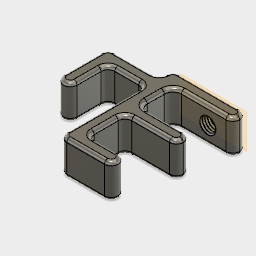
Clamp-Hooks (Autodesk Fusion 360 design; units mm, degrees)
Autodesk Fusion 360 part; units mm, degrees
sketch "Sketch1" plane through (0, 0, 0) normal (0, 1, 0) x (1, 0, 0)
  line L0 (-5, 15) -> (30, 15)
  line L1 (30, 15) -> (30, -5)
  line L2 (30, -5) -> (-5, -5)
  line L3 (-5, -5) -> (-5, 15)
  line L4 (30, 23) -> (-13, 23)
  line L5 (-13, 23) -> (-13, -13)
  line L6 (-13, -13) -> (30, -13)
  line L7 (30, -13) -> (30, 23)
  line L8 (-13, -13) -> (-49, -13)
  line L9 (-49, -13) -> (-49, 23)
  line L10 (-49, 23) -> (-13, 23)
  line L11 (-13, 23) -> (-13, -13)
  line L12 (30, -5) -> (25, -5)
  line L13 (25, -5) -> (25, -13)
  line L14 (25, -13) -> (30, -13)
  line L15 (30, -13) -> (30, -5)
  dimension "d7" = 36
  dimension "d21" = 8
  dimension "d22" = 5
  constraint horizontal L0
  constraint vertical L1
  constraint horizontal L2
  constraint vertical L3
  constraint horizontal L4
  constraint vertical L5
  constraint horizontal L6
  constraint vertical L7
  constraint horizontal L8
  constraint vertical L9
  constraint horizontal L10
  constraint vertical L11
  constraint horizontal L12
  constraint vertical L13
  constraint horizontal L14
  constraint vertical L15
  measures "d7" distance of origin
  measures "d21" distance of origin
extrude "Extrude1" add sketch "Sketch1" along normal blind 20 contours L0 L2 L3 L4 L5 L6 L7 L11 L13 | L2 L6 L7 L12 L13 L14 L15
fillet "Fillet2" radius 5 2 edges at (-5, 10, 5) (-5, 10, -15)
sketch "Sketch2" plane through (0, 0, -15) normal (0, 0, 1) x (1, 0, 0)
  line L0 (0, 20) -> (0, 0)
  line L1 (0, 0) -> (30, 0)
  line L2 (30, 0) -> (30, 20)
  line L3 (30, 20) -> (0, 20)
  circle A0 centre (15, 10) radius 5
extrude "Extrude2" cut sketch "Sketch2" against normal blind 10 contours A0
thread "Thread1" "ISO Metric profile 10.0 M10x1.5 6H" major diameter 10.198 minor diameter 8.526 pitch 1.5 angle 60 modelled right hand crest width 0.1875 on face at (19.9752, 9.5022, -17.6667) crest through (19.263, 10, -14.1562)
sketch "Sketch5" plane through (0, 0, 0) normal (0, -1, 0) x (1, 0, 0)
  line L0 (30, 5) -> (30, 13)
  line L1 (30, 13) -> (-13, 13)
  line L2 (-13, 13) -> (-13, -23)
  line L3 (-13, -23) -> (30, -23)
  line L4 (30, -23) -> (30, -15)
  line L5 (30, -15) -> (0, -15)
  arc A0 (-5, -10) -> (0, -15) centre (0, -10) ccw
  line L6 (-5, -10) -> (-5, 0)
  arc A1 (0, 5) -> (-5, 0) centre (0, 0) ccw
  line L7 (0, 5) -> (30, 5)
  line L8 (-13, -15) -> (-43, -15)
  line L9 (-43, -15) -> (-43, 15)
  line L10 (-43, 15) -> (-13, 15)
  line L11 (-13, 15) -> (-13, -15)
  line L12 (-13, 15) -> (-35, 15)
  line L13 (-35, 15) -> (-35, -7)
  line L14 (-35, -7) -> (-13, -7)
  line L15 (-13, -7) -> (-13, 15)
  line L16 (-13, 13) -> (17, 13)
  line L17 (17, 13) -> (17, 43)
  line L18 (17, 43) -> (-13, 43)
  line L19 (-13, 43) -> (-13, 13)
  line L20 (17, 13) -> (-5, 13)
  line L21 (-5, 13) -> (-5, 35)
  line L22 (-5, 35) -> (17, 35)
  line L23 (17, 35) -> (17, 13)
  dimension "d10" = 30
  dimension "d11" = 30
  dimension "d12" = 22
  dimension "d13" = 22
  dimension "d14" = 30
  dimension "d15" = 30
  dimension "d16" = 22
  dimension "d17" = 22
  constraint horizontal L8
  constraint vertical L9
  constraint horizontal L10
  constraint vertical L11
  constraint coincident L2 A1.centre
  constraint horizontal L12
  constraint vertical L13
  constraint horizontal L14
  constraint vertical L15
  constraint horizontal L16
  constraint vertical L17
  constraint horizontal L18
  constraint vertical L19
  constraint horizontal L20
  constraint vertical L21
  constraint horizontal L22
  constraint vertical L23
  measures "d12" distance of A1.centre
  measures "d14" distance of A1.centre
  measures "d17" distance of A1.centre
extrude "Extrude3" add sketch "Sketch5" against normal blind 20 contours L1 L11 L15 L16 L17 L18 L19 L21 L22 | L2 L8 L9 L10 L11 L13 L14
fillet "Fillet3" radius 4 10 edges at (-13, 10, -23) (-43, 10, -15) (-13, 10, 43) (-13, 10, -7) (-35, 10, -7) (-13, 10, -15) (-43, 10, 15) (-35, 10, 15) (17, 10, 43) (17, 10, 35)
sketch "Sketch6" plane through (0, 20, 0) normal (0, 1, 0) x (-1, 0, 0)
  arc A0 (-13, 43) -> (-13, 35) centre (-13, 39) ccw
  line L0 (-13, 35) -> (5, 35)
  line L1 (5, 35) -> (5, 13)
  line L2 (5, 13) -> (-30, 13)
  line L3 (-30, 13) -> (-30, 5)
  line L4 (-30, 5) -> (0, 5)
  arc A1 (5, 0) -> (0, 5) centre (0, 0) ccw
  line L5 (5, 0) -> (5, -10)
  arc A2 (0, -15) -> (5, -10) centre (0, -10) ccw
  line L6 (0, -15) -> (-30, -15)
  line L7 (-30, -15) -> (-30, -23)
  line L8 (-30, -23) -> (9, -23)
  arc A3 (9, -23) -> (13, -19) centre (9, -19) ccw
  arc A4 (17, -15) -> (13, -19) centre (17, -19) ccw
  line L9 (17, -15) -> (39, -15)
  arc A5 (39, -15) -> (43, -11) centre (39, -11) ccw
  line L10 (43, -11) -> (43, 11)
  arc A6 (43, 11) -> (35, 11) centre (39, 11) ccw
  line L11 (35, 11) -> (35, -3)
  arc A7 (31, -7) -> (35, -3) centre (31, -3) ccw
  line L12 (31, -7) -> (17, -7)
  arc A8 (13, -3) -> (17, -7) centre (17, -3) ccw
  line L13 (13, -3) -> (13, 39)
  arc A9 (13, 39) -> (9, 43) centre (9, 39) ccw
  line L14 (9, 43) -> (-13, 43)
  line L15 (-30, 5) -> (-25, 5)
  line L16 (-25, 5) -> (-25, 13)
  line L17 (-25, 13) -> (-30, 13)
  line L18 (-30, 13) -> (-30, 5)
  dimension "d23" = 5
  constraint horizontal L15
  constraint vertical L16
  constraint horizontal L17
  constraint vertical L18
  constraint coincident A1.centre origin
extrude "Extrude4" cut sketch "Sketch6" against normal blind 20 contours L2 L3 L4 L15 L16 L17 L18
sketch "Sketch7" plane through (0, 0, -23) normal (0, 0, -1) x (-1, 0, 0)
  line L0 (9, 0) -> (9, 20)
  line L1 (9, 20) -> (-30, 20)
  line L2 (-30, 20) -> (-30, 0)
  line L3 (-30, 0) -> (9, 0)
  spline S0 degree 3 poles (-14.0411, 4.992) (-14.689, 4.9215) (-15.3444, 4.9764) (-16.5762, 5.3323) (-17.1429, 5.6222) (-18.1146, 6.3932) (-18.5151, 6.8606) (-19.1008, 7.9064) (-19.2872, 8.4709) (-19.4007, 9.404) (-19.4016, 9.7566) (-19.3193, 10.4465) (-19.2383, 10.7817) (-19.1177, 11.1033) knots 0 0 0 0 0.195529 0.195529 0.384922 0.384922 0.568175 0.568175 0.745285 0.745285 0.850991 0.850991 0.954382 0.954382 0.954382 0.954382
  arc A0 (-17.1315, 13.6919) -> (-19.1177, 11.1033) centre (-15, 10) ccw
  spline S1 degree 3 poles (-17.1315, 13.6919) (-16.6737, 14.0189) (-16.1555, 14.2517) (-15.0394, 14.5142) (-14.4506, 14.5337) (-13.2771, 14.3464) (-12.7051, 14.1336) (-11.6549, 13.4932) (-11.191, 13.065) (-10.5862, 12.2422) (-10.3915, 11.8962) (-10.0851, 11.1584) (-9.9761, 10.7686) (-9.9144, 10.3699) knots 0 0 0 0 0.168783 0.168783 0.343691 0.343691 0.524721 0.524721 0.711872 0.711872 0.830165 0.830165 0.950778 0.950778 0.950778 0.950778
  arc A1 (-14.0411, 4.992) -> (-9.9144, 10.3699) centre (-15, 10) ccw
fillet "Fillet4" radius 4 5 edges at (-5, 10, 13) (25, 10, 13) (25, 10, 5) (30, 10, -15) (30, 10, -23)
fillet "Fillet5" radius 4 1 edges at (-5, 10, 35)
fillet "Fillet6" radius 2 29 edges at (-43, 20, 0) (-41.8284, 20, -13.8284) (-28, 20, -15) (-14.1716, 20, -16.1716) (-11.8284, 20, -21.8284) (8.5, 20, -23) (28.8284, 20, -21.8284) (28.8284, 20, -16.1716) (13, 20, -15) (-3.5355, 20, -13.5355) (-5, 20, -5) (-3.5355, 20, 3.5355) (10.5, 20, 5) (23.8284, 20, 6.1716) (23.8284, 20, 11.8284) (10, 20, 13) (-3.8284, 20, 14.1716) (-5, 20, 24) (-3.8284, 20, 33.8284) (6, 20, 35) (17, 20, 39) (2, 20, 43) (-11.8284, 20, 41.8284) (-13, 20, 18) (-14.1716, 20, -5.8284) (-24, 20, -7) (-33.8284, 20, -5.8284) (-35, 20, 4) (-39, 20, 15)
fillet "Fillet7" radius 2 29 edges at (-33.8284, 0, -5.8284) (-24, 0, -7) (-14.1716, 0, -5.8284) (-13, 0, 18) (-11.8284, 0, 41.8284) (2, 0, 43) (17, 0, 39) (6, 0, 35) (-3.8284, 0, 33.8284) (-5, 0, 24) (-3.8284, 0, 14.1716) (10, 0, 13) (23.8284, 0, 11.8284) (23.8284, 0, 6.1716) (10.5, 0, 5) (-3.5355, 0, 3.5355) (-5, 0, -5) (-3.5355, 0, -13.5355) (13, 0, -15) (28.8284, 0, -16.1716) (28.8284, 0, -21.8284) (8.5, 0, -23) (-11.8284, 0, -21.8284) (-14.1716, 0, -16.1716) (-28, 0, -15) (-41.8284, 0, -13.8284) (-43, 0, 0) (-39, 0, 15) (-35, 0, 4)
sketch "Sketch3" plane through (0, 0, 0) normal (0, -1, 0) x (1, 0, 0)
  line L0 (25, 5) -> (25, 13)
  line L1 (25, 13) -> (-13, 13)
  line L2 (-13, 13) -> (-13, -23)
  line L3 (-13, -23) -> (25, -23)
  line L4 (25, -23) -> (25, -15)
  line L5 (25, -15) -> (0, -15)
  arc A0 (-5, -10) -> (0, -15) centre (0, -10) ccw
  line L6 (-5, -10) -> (-5, 0)
  arc A1 (0, 5) -> (-5, 0) centre (0, 0) ccw
  line L7 (0, 5) -> (25, 5)
  line L8 (-13, 13) -> (-49, 13)
  line L9 (-49, 13) -> (-49, -23)
  line L10 (-49, -23) -> (-13, -23)
  line L11 (-13, -23) -> (-13, 13)
  line L12 (-13, 13) -> (-40, 13)
  line L13 (-40, 13) -> (-40, -15)
  line L14 (-40, -15) -> (-13, -15)
  line L15 (-13, -15) -> (-13, 13)
  dimension "d8" = 36
  dimension "d9" = 36
  constraint horizontal L8
  constraint vertical L9
  constraint horizontal L10
  constraint vertical L11
  constraint horizontal L12
  constraint vertical L13
  constraint horizontal L14
  constraint vertical L15
sketch "Sketch4" plane through (0, 0, 0) normal (0, 1, 0) x (1, 0, 0)
